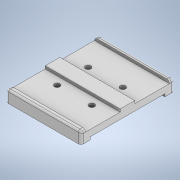
# Autodesk Inventor part: base
Saved by Autodesk Inventor 2021 (Build 250183000, 183)
## iProperties
Created: 2022-04-24
Part Number: base
Material: Generic
Document SubType Name: Modeling
Designer: hp
Density: 1 g/cm^3
Appearance: Default
Author: hp
Autodesk Inventor part; units mm, degrees
ref_plane "YZ Plane" through (0, 0, 0) normal (1, 0, 0) x (0, 1, 0)
ref_plane "XZ Plane" through (0, 0, 0) normal (0, 1, 0) x (-1, 0, 0)
ref_plane "XY Plane" through (0, 0, 0) normal (0, 0, 1) x (1, 0, 0)
sketch "Sketch1" plane through (0, 0, 0) normal (1, 0, 0) x (0, 1, 0)
  line L0 (7, 51) -> (0, 51)
  line L1 (0, 41) -> (0, -41)
  line L2 (0, -51) -> (7, -51)
  line L3 (7, 51) -> (-3, 51)
  line L4 (-3, 51) -> (-3, 41)
  line L5 (-3, 41) -> (0, 41)
  line L6 (7, 41) -> (7, 51)
  line L7 (7, 51) -> (8, 51)
  line L8 (10, 49) -> (10, 46)
  line L9 (10, 46) -> (7, 46)
  line L10 (7, 46) -> (7, 51)
  line L11 (7, 8) -> (10, 8)
  line L12 (10, 8) -> (10, -8)
  line L13 (10, -8) -> (7, -8)
  line L14 (7, 0) -> (0, 0)
  line L15 (7, -51) -> (0, -51)
  line L16 (7, -51) -> (-3, -51)
  line L17 (-3, -51) -> (-3, -41)
  line L18 (-3, -41) -> (0, -41)
  line L19 (7, -41) -> (7, -46)
  line L20 (7, -51) -> (7, -51)
  line L21 (10, -48) -> (10, -46)
  line L22 (10, -46) -> (7, -46)
  line L23 (7, -46) -> (7, -8)
  line L24 (7, 8) -> (7, 51)
  arc A0 (10, 49) -> (8, 51) centre (8, 49) ccw
  arc A1 (7, -51) -> (10, -48) centre (7, -48) ccw
  point P0 (10, 51)
  point P1 (10, -51)
  point P2 (0, 51)
  dimension "d0" = 102
  dimension "d1" = 51
  dimension "d2" = 3
  dimension "d3" = 5
  dimension "d4" = 3
  dimension "d6" = 43
  dimension "d7" = 59
  dimension "d9" = 10
  dimension "d10" = 2
  dimension "d11" = 3
  constraints: 50 end point, 8 parallel, 6 symmetric about line, 4 horizontal, 4 perpendicular, 4 point on circle, 4 point on line, 4 tangent, 2 centre point
  measures "d0" distance of L0.end L2.start
  measures "d1" distance from line of L0 L14.end
  measures "d2" distance between parallel lines of L4 L1
  measures "d3" distance of point (10, 51) L8.end
  measures "d4" distance of L0.start point (10, 51)
  measures "d6" distance between parallel lines of L7 L11
  measures "d7" distance between parallel lines of L7 L13
  measures "d9" distance of L3.end L4.end
  measures "d10" radius of A0
  measures "d11" radius of A1
extrude "Extrusion1" add sketch "Sketch1" along normal blind 82
fillet "Fillet1" radius 3 9 edges at (82, 9.4142, 50.4142) (82, 10, 47.5) (82, -1.5, 51) (82, 3.5, 51) (82, 7.5, 51) (82, 9.1213, -50.1213) (82, 10, -47) (82, 3.5, -51) (82, -1.5, -51)
fillet "Fillet2" radius 3 6 edges at (0, 9.1213, -50.1213) (0, 10, -47) (0, 2, -51) (0, 9.4142, 50.4142) (0, 10, 47.5) (0, 2.5, 51)
sketch "Sketch2" plane through (0, 7, 8) normal (0, 1, 0) x (1, 0, 0)
  circle A0 centre (22, -9) radius 3
  line L0 (0, 0) -> (0, -38) projected
  line L1 (3, -43) -> (79, -43) projected
  circle A1 centre (60, -9) radius 3
  circle A2 centre (60, 25) radius 3
  circle A3 centre (22, 25) radius 3
  line L2 (3, 59) -> (79, 59) projected
  line L3 (0, 54) -> (0, 16) projected
  line L4 (82, 0) -> (82, -38) projected
  line L5 (82, 54) -> (82, 16) projected
  point P0 (0, 8)
  dimension "d16" = 6
  dimension "d17" = 22
  dimension "d18" = 34
  dimension "d19" = 6
  dimension "d20" = 6
  dimension "d21" = 6
  dimension "d22" = 34
  dimension "d23" = 34
  dimension "d24" = 34
  dimension "d25" = 22
  dimension "d26" = 22
  dimension "d27" = 22
  constraints: 4 centre point
  measures "d16" diameter of A0
  measures "d17" distance from line of L0 A0.centre
  measures "d18" distance from line of L1 A0.centre
  measures "d19" diameter of A3
  measures "d20" diameter of A2
  measures "d21" diameter of A1
  measures "d22" distance from line of L1 A1.centre
  measures "d23" distance from line of L2 A2.centre
  measures "d24" distance from line of L2 A3.centre
  measures "d25" distance from line of L3 A3.centre
  measures "d26" distance from line of L4 A1.centre
  measures "d27" distance from line of L5 A2.centre
extrude "Extrusion2" cut sketch "Sketch2" against normal blind 82
equation "\"d1\" = 0.5 * d0"
equation "\"d19\" = d16"
equation "\"d20\" = d16"
equation "\"d21\" = d16"
equation "\"d22\" = d18"
equation "\"d23\" = d18"
equation "\"d24\" = d18"
equation "\"d25\" = d17"
equation "\"d26\" = d17"
equation "\"d27\" = d25"
body "Solid1"
